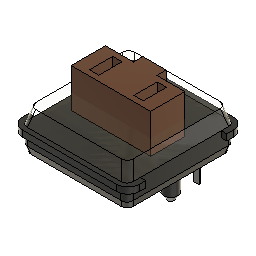
Choc v1 v9 (Autodesk Fusion 360 design; units mm, degrees)
Autodesk Fusion 360 part; units mm, degrees
sketch "Body" plane through (0, 0, 0) normal (0, 0, 1) x (1, 0, 0)
  line L0 (6.8, -6.9) -> (-6.8, -6.9)
  line L1 (-6.8, -6.9) -> (-6.8, 6.9)
  line L2 (-6.8, 6.9) -> (6.8, 6.9)
  line L3 (6.8, 6.9) -> (6.8, -6.9)
  line L4 (6.8, -6.9) -> (-6.8, 6.9) construction
  line L5 (-6.8, -6.9) -> (6.8, 6.9) construction
  line L6 (7.5, -7.5) -> (-7.5, -7.5)
  line L7 (-7.5, -7.5) -> (-7.5, 7.5)
  line L8 (-7.5, 7.5) -> (7.5, 7.5)
  line L9 (7.5, 7.5) -> (7.5, -7.5)
  line L10 (7.5, -7.5) -> (-7.5, 7.5) construction
  line L11 (-7.5, -7.5) -> (7.5, 7.5) construction
  line L12 (-7.5, 5.2) -> (-6.8, 5.2)
  line L13 (0, 2.5) -> (0, 20)
  line L14 (7.5, 5.2) -> (6.8, 5.2)
  line L15 (20, 0) -> (2.5, 0)
  line L16 (-7.5, -5.2) -> (-6.8, -5.2)
  line L17 (7.5, -5.2) -> (6.8, -5.2)
  circle A0 centre (0, 0) radius 1.6
  circle A1 centre (5.5, 0) radius 0.9
  line L18 (0, 1.75) -> (0, 22.5)
  circle A2 centre (-5.5, 0) radius 0.9
  line L19 (0.4, 5.85) -> (-0.4, 5.85)
  line L20 (-0.4, 5.85) -> (-0.4, 5.95)
  line L21 (-0.4, 5.95) -> (0.4, 5.95)
  line L22 (0.4, 5.95) -> (0.4, 5.85)
  line L23 (0.4, 5.85) -> (-0.4, 5.95) construction
  line L24 (-0.4, 5.85) -> (0.4, 5.95) construction
  line L25 (5.4, 3.75) -> (4.6, 3.75)
  line L26 (4.6, 3.75) -> (4.6, 3.85)
  line L27 (4.6, 3.85) -> (5.4, 3.85)
  line L28 (5.4, 3.85) -> (5.4, 3.75)
  line L29 (5.4, 3.75) -> (4.6, 3.85) construction
  line L30 (4.6, 3.75) -> (5.4, 3.85) construction
  line L31 (1.75, 0) -> (22.5, 0)
  line L32 (-7.5, 1.75) -> (-6.8, 1.75)
  line L33 (7.5, 1.75) -> (6.8, 1.75)
  line L34 (-7.5, -1.75) -> (-6.8, -1.75)
  line L35 (7.5, -1.75) -> (6.8, -1.75)
  line L36 (9.5, -9.5) -> (-9.5, -9.5)
  line L37 (-9.5, -9.5) -> (-9.5, 9.5)
  line L38 (-9.5, 9.5) -> (9.5, 9.5)
  line L39 (9.5, 9.5) -> (9.5, -9.5)
  line L40 (9.5, -9.5) -> (-9.5, 9.5) construction
  line L41 (-9.5, -9.5) -> (9.5, 9.5) construction
  point P0 (0, 5.9)
  point P1 (5, 3.8)
  dimension "d1" = 13.6
  dimension "d2" = 13.8
  dimension "d3" = 15
  dimension "d4" = 2.3
  dimension "d5" = 3.2
  dimension "d6" = 1.8
  dimension "d7" = 5.5
  dimension "d29" = 5.9
  dimension "d30" = 0.1
  dimension "d31" = 0.8
  dimension "d32" = 5
  dimension "d33" = 3.8
  dimension "d34" = 0.1
  dimension "d35" = 0.8
  dimension "d85" = 1.75
  dimension "Pitch" = 19
  constraint horizontal L0
  constraint perpendicular L0 L1
  constraint parallel L0 L2
  constraint parallel L1 L3
  constraint coincident L4 A0.centre
  constraint coincident L5 A0.centre
  constraint coincident A0.centre origin
  constraint horizontal L6
  constraint perpendicular L6 L7
  constraint parallel L6 L8
  constraint parallel L7 L9
  constraint coincident L10 A0.centre
  constraint coincident L11 A0.centre
  constraint equal L8 L9
  constraint coincident L7 L12.start
  constraint coincident L1 L12.end
  constraint perpendicular L1 L12
  constraint symmetric L12.start L13 L14.start
  constraint symmetric L12.end L13 L14.end
  constraint symmetric L12.start L15 L16.start
  constraint symmetric L12.end L15 L16.end
  constraint symmetric L14.start L15 L17.start
  constraint symmetric L14.end L15 L17.end
  constraint coincident L15 A1.centre
  constraint symmetric L13 A1 A2
  constraint horizontal L19
  constraint perpendicular L19 L20
  constraint parallel L19 L21
  constraint parallel L20 L22
  constraint coincident L23 P0
  constraint coincident L24 P0
  constraint coincident L18 P0
  constraint horizontal L25
  constraint perpendicular L25 L26
  constraint parallel L25 L27
  constraint parallel L26 L28
  constraint coincident L29 P1
  constraint coincident L30 P1
  constraint coincident L7 L32.start
  constraint coincident L1 L32.end
  constraint perpendicular L1 L32
  constraint symmetric L13 L32.start L33.start
  constraint symmetric L13 L32.end L33.end
  constraint symmetric L15 L32.start L34.start
  constraint symmetric L15 L32.end L34.end
  constraint symmetric L15 L33.start L35.start
  constraint symmetric L15 L33.end L35.end
  constraint horizontal L36
  constraint perpendicular L36 L37
  constraint parallel L36 L38
  constraint parallel L37 L39
  constraint coincident L40 A0.centre
  constraint coincident L41 A0.centre
  constraint equal L37 L38
  measures "d1" distance of L0.start L0.end
  measures "d2" distance of L0.start L2.end
  measures "d3" distance of L6.start L6.end
  measures "d4" distance of L8 L12
  measures "d5" diameter of A0
  measures "d6" diameter of A1
  measures "d7" distance of A1.centre L18
  measures "d29" distance of A0.centre P0
  measures "d30" distance of L19.start L21.end
  measures "d31" distance of L19.start L19.end
  measures "d32" horizontal distance of A0.centre P1
  measures "d33" distance of P1 L31
  measures "d34" distance of L25.end L26.end
  measures "d35" distance of L25.start L25.end
  measures "d85" distance of A0.centre L32
  measures "Pitch" distance of L37.end L38.end
ref_plane "WorkPlane1" through (0, 0, 0.8) normal (0, 0, 1) x (1, 0, 0)
ref_plane "WorkPlane2" through (0, 0, 2.8) normal (0, 0, 1) x (1, 0, 0)
ref_plane "WorkPlane3" through (0, 0, -2.2) normal (0, 0, 1) x (1, 0, 0)
ref_plane "WorkPlane4" through (0, 0, -1.3) normal (0, 0, 1) x (1, 0, 0)
extrude "Extrude1" add sketch "Body" along normal up to surface (2 mm away) draft -15 from surface at 0.8 contours L0 L1 L2 L3 | L13 L18 L19 L20 L21 | L13 L18 L19 L21 L22 | L15 A1 L31 | L15 A1 L31 | A0 | A2 | L25 L26 L27 L28 makes body 1
extrude "Extrude2" add sketch "Body" along normal up to surface (0.8 mm away) separate body contours L0 L1 L3 L6 L7 L9 L16 L17 | L0 L1 L2 L3 | L1 L2 L7 L8 L12 L13 L18 | L2 L3 L8 L9 L13 L14 L18 | L13 L18 L19 L20 L21 | L13 L18 L19 L21 L22 | L15 A1 L31 | L15 A1 L31 | A0 | A2 | L25 L26 L27 L28 makes body 2
extrude "Extrude3" add sketch "Body" against normal up to surface (1.3 mm away) contours L0 L1 L2 L3 | L13 L18 L19 L20 L21 | L13 L18 L19 L21 L22 | L15 A1 L31 | L15 A1 L31 | A0 | A2 | L25 L26 L27 L28 bodies 2
extrude "Extrude4" add sketch "Body" against normal up to surface (0.9 mm away) draft -15 from surface at -1.3 contours L0 L1 L2 L3 | L13 L18 L19 L20 L21 | L13 L18 L19 L21 L22 | L15 A1 L31 | L15 A1 L31 | A0 | A2 | L25 L26 L27 L28 bodies 2
extrude "Extrude5" add sketch "Body" against normal blind 2.65 from surface at -2.2 contours L15 A1 L31 | L15 A1 L31 | A0 | A2 bodies 2
chamfer "Chamfer1" distance 0.5 distance2 0.8 2 edges at (4.6609, 0.3255, -4.85) (-6.3391, 0.3255, -4.85) measured on face at (5.2164, -0.0417, -4.85) measured on face at (-5.7836, -0.0417, -4.85) on bodies 2
chamfer "Chamfer2" distance 0.5 distance2 1 1 edges at (-1.4917, 0.5786, -4.85) measured on face at (0.5957, -0.3358, -4.85) on bodies 2
extrude "Extrude6" add sketch "Body" against normal blind 3 from surface at -2.2 separate body contours L13 L18 L19 L20 L21 | L13 L18 L19 L21 L22 | L25 L26 L27 L28 makes body 3 at (-0.1333, 5.95, -3.2) makes body 4 at (5.1333, 3.75, -4.2)
sketch "Stem" plane through (0, 0, 2.8) normal (0, 0, 1) x (1, 0, 0)
  line L0 (5.1, -2.2) -> (-5.1, -2.2)
  line L1 (-5.1, -2.2) -> (-5.1, 2.2)
  line L2 (-5.1, 2.2) -> (5.1, 2.2)
  line L3 (5.1, 2.2) -> (5.1, -2.2)
  line L4 (5.1, -2.2) -> (-5.1, 2.2) construction
  line L5 (-5.1, -2.2) -> (5.1, 2.2) construction
  line L6 (1.5, 2.2) -> (-1.5, 2.2)
  line L7 (-1.5, 2.2) -> (-1.5, 3.4)
  line L8 (-1.5, 3.4) -> (1.5, 3.4)
  line L9 (1.5, 3.4) -> (1.5, 2.2)
  line L10 (1.5, 2.2) -> (-1.5, 3.4) construction
  line L11 (-1.5, 2.2) -> (1.5, 3.4) construction
  line L12 (0, 1.75) -> (0, 22.5)
  line L13 (-2.25, -1.5) -> (-3.45, -1.5)
  line L14 (-3.45, -1.5) -> (-3.45, 1.5)
  line L15 (-3.45, 1.5) -> (-2.25, 1.5)
  line L16 (-2.25, 1.5) -> (-2.25, -1.5)
  line L17 (-2.25, -1.5) -> (-3.45, 1.5) construction
  line L18 (-3.45, -1.5) -> (-2.25, 1.5) construction
  line L19 (1.75, 0) -> (22.5, 0)
  line L20 (0, 2.5) -> (0, 20)
  line L21 (3.45, 1.5) -> (2.25, 1.5)
  line L22 (2.25, 1.5) -> (2.25, -1.5)
  line L23 (2.25, -1.5) -> (3.45, -1.5)
  line L24 (3.45, -1.5) -> (3.45, 1.5)
  point P0 (0, 2.8)
  point P1 (-2.85, 0)
  dimension "d39" = 4.4
  dimension "d40" = 10.2
  dimension "d41" = 1.2
  dimension "d42" = 3
  dimension "d43" = 1.2
  dimension "d44" = 3
  dimension "d45" = 5.7
  constraint horizontal L0
  constraint perpendicular L0 L1
  constraint parallel L0 L2
  constraint parallel L1 L3
  constraint coincident L4 origin
  constraint coincident L5 origin
  constraint horizontal L6
  constraint perpendicular L6 L7
  constraint parallel L6 L8
  constraint parallel L7 L9
  constraint coincident L2 L6.start
  constraint coincident L10 P0
  constraint coincident L11 P0
  constraint coincident P0 L12
  constraint horizontal L13
  constraint perpendicular L13 L14
  constraint parallel L13 L15
  constraint parallel L14 L16
  constraint coincident L17 P1
  constraint coincident L18 P1
  constraint coincident P1 L19
  constraint symmetric L13.start L20 L22.end
  constraint symmetric L13.end L20 L23.end
  constraint symmetric L14.end L20 L21.start
  constraint symmetric L15.end L20 L21.end
  measures "d39" distance of L0.start L2.end
  measures "d40" distance of L0.start L0.end
  measures "d41" distance of L6.start L8.end
  measures "d42" distance of L7.end L8.end
  measures "d43" distance of L14.end L15.end
  measures "d44" distance of L13.end L14.end
  measures "d45" distance of L15.end L21.start
extrude "Extrude7" add sketch "Stem" along normal blind 3 and the other way up to surface (2 mm away) separate body makes body 5
fillet "Fillet1" radius 1.5 4 edges at (7.5, -7.5, 0.4) (-7.5, -7.5, 0.4) (-7.5, 7.5, 0.4) (7.5, 7.5, 0.4) on bodies 2
fillet "Fillet2" radius 0.8 8 edges at (6.8, 6.9, -0.65) (6.6794, 6.7794, -1.75) (6.8, -6.9, -0.65) (6.6794, -6.7794, -1.75) (-6.8, -6.9, -0.65) (-6.6794, -6.7794, -1.75) (-6.8, 6.9, -0.65) (-6.6794, 6.7794, -1.75) on bodies 2
fillet "Fillet3" radius 0.8 4 edges at (6.5321, -6.6321, 1.8) (-6.5321, -6.6321, 1.8) (6.5321, 6.6321, 1.8) (-6.5321, 6.6321, 1.8) on bodies 1
extrude "Extrude8" add sketch "Body" against normal up to surface (2.2 mm away) separate body contours L0 L1 L2 L3 | L13 L18 L19 L20 L21 | L13 L18 L19 L21 L22 | L15 A1 L31 | L15 A1 L31 | A0 | A2 | L25 L26 L27 L28 makes body 6
extrude "Extrude9" add sketch "Body" along normal blind 10 contours L0 L1 L3 L6 L7 L9 L16 L17 | L0 L1 L2 L3 | L3 L9 L17 L35 | L1 L7 L16 L34 | L3 L9 L15 L31 L35 | L6 L7 L8 L9 L13 L15 L18 L31 L36 L37 L38 L39 | L1 L7 L32 L34 | L3 L9 L15 L31 L33 | L1 L7 L12 L32 | L3 L9 L14 L33 | L8 L9 L13 L15 L18 L31 L38 L39 | L1 L2 L7 L8 L12 L13 L18 | L2 L3 L8 L9 L13 L14 L18 | L13 L18 L19 L20 L21 | L13 L18 L19 L21 L22 | L15 A1 L31 | L15 A1 L31 | A0 | A2 | L25 L26 L27 L28 bodies 6
fillet "Fillet4" radius 0.7 4 edges at (6.8, -6.9, -1.1) (-6.8, -6.9, -1.1) (-6.8, 6.9, -1.1) (6.8, 6.9, -1.1) on bodies 6
fillet "Fillet5" radius 1 4 edges at (9.5, -9.5, 5) (-9.5, -9.5, 5) (-9.5, 9.5, 5) (9.5, 9.5, 5) on bodies 6
extrude "Extrude10" add sketch "Body" against normal up to surface (0.9 mm away) from surface at -1.3 contours L3 L9 L17 L35 | L1 L7 L16 L34 | L1 L7 L12 L32 | L3 L9 L14 L33 bodies 6
extrude "Extrude11" add sketch "Body" against normal up to surface (1.3 mm away) separate body contours L0 L1 L3 L6 L7 L9 L16 L17 | L3 L9 L17 L35 | L1 L7 L16 L34 | L3 L9 L15 L31 L35 | L1 L7 L32 L34 | L3 L9 L15 L31 L33 | L1 L7 L12 L32 | L3 L9 L14 L33 | L1 L2 L7 L8 L12 L13 L18 | L2 L3 L8 L9 L13 L14 L18 makes body 7
fillet "Fillet6" radius 0.7 4 edges at (6.8, -6.9, -0.65) (-6.8, -6.9, -0.65) (-6.8, 6.9, -0.65) (6.8, 6.9, -0.65) on bodies 7
sketch "Hole" plane through (0, 0, 0) normal (0, 0, 1) x (1, 0, 0)
  line L0 (11, -12) -> (-11, -12)
  line L1 (-12, -11) -> (-12, 11)
  line L2 (-11, 12) -> (11, 12)
  line L3 (12, 11) -> (12, -11)
  line L4 (12, -12) -> (-12, 12) construction
  line L5 (-12, -12) -> (12, 12) construction
  line L6 (28, -5) -> (28, -9)
  arc A0 (12, 11) -> (11, 12) centre (11, 11) ccw
  arc A1 (11, -12) -> (12, -11) centre (11, -11) ccw
  arc A2 (-12, -11) -> (-11, -12) centre (-11, -11) ccw
  arc A3 (-11, 12) -> (-12, 11) centre (-11, 11) ccw
  dimension "PitchMargin" = 4
  dimension "BridgeR" = 1
  dimension "d77" = 24
  dimension "d78" = 24
  constraint horizontal L0
  constraint perpendicular L0 L1
  constraint parallel L0 L2
  constraint parallel L1 L3
  constraint coincident L4 origin
  constraint coincident L5 origin
  constraint perpendicular L2 L6
  constraint coincident L5.end L2
  constraint coincident L5.end L3
  constraint tangent L2 A0
  constraint tangent L3 A0
  constraint coincident L4.start L3
  constraint coincident L4.start L0
  constraint tangent L3 A1
  constraint tangent L0 A1
  constraint equal A0 A1
  constraint coincident L5.start L0
  constraint coincident L5.start L1
  constraint tangent L0 A2
  constraint tangent L1 A2
  constraint equal A0 A2
  constraint coincident L4.end L1
  constraint coincident L4.end L2
  constraint tangent L1 A3
  constraint tangent L2 A3
  constraint equal A0 A3
  measures "PitchMargin" distance of L6.start L6.end
  measures "BridgeR" radius of A0
  measures "d77" distance of L1 L3
  measures "d78" distance of L0 L2
extrude "Extrude12" add sketch "Hole" against normal blind 7 separate body makes body 8
copy_body "CopyPasteBodies1" bodies 2 makes body 9
combine "Combine1" operation add target body 9 tool bodies 1 keep tools
copy_body "CopyPasteBodies2" bodies 8 makes body 10
combine "Combine2" operation add target body 10 tool bodies 6 keep tools
move_body "Move1" bodies 1 5 2 3 4 6 7 8 9 10 to x (1, 0, 0) y (0, 1, 0) z (0, 0, 1) at (0, 0, 0)
move_body "Move2" bodies 1 5 2 3 4 6 7 8 9 10 to x (1, 0, 0) y (0, 1, 0) z (0, 0, 1) at (0, 0, 0)
hidden bodies 6 7 8 9 10
equation "d77 = Pitch + PitchMargin + BridgeR"
equation "d78 = Pitch + PitchMargin + BridgeR"
equation "SwitchAngle = 0.0 deg"
equation "SwitchX = 0.00 mm"
equation "SwitchY = 0.00 mm"
equation "d88 = BridgeR"
named bodies: "Upper", "Lower", "Terminal1", "Terminal2", "Stem", "Hole", "MF", "Fill", "MEV", "Territory"
